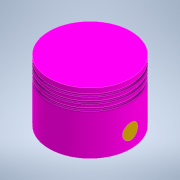
# Autodesk Inventor part: Piston
Saved by Autodesk Inventor 2021 (Build 250183000, 183)
## iProperties
Created: 2021-04-09
Part Number: Piston
Material: Aluminum 6061
Document SubType Name: Modeling
Designer: tommy
Density: 2.7 g/cm^3
Appearance: Magenta
Mass: 463.137 g
Surface Area: 642.196 cm^2
Volume: 171.532 cm^3
bore_dia: 4.000 in
piston_height: 3.000 in
d3: 0.00 deg
wall_thick: 0.250 in
d6: 2.750 in
d7: 0.00 deg
pin_dia: 0.750 in
d11: 1.500 in
d12: 0.750 in
d14: 0.00 deg
ring_depth: 0.100 in
ring_height: 0.150 in
ring_offset: 0.250 in
d19: 3.000 ul
ring_spacing: 0.300 in
Author: tommy
Autodesk Inventor part; units mm, degrees
ref_plane "YZ Plane" through (0, 0, 0) normal (1, 0, 0) x (0, 1, 0)
ref_plane "XZ Plane" through (0, 0, 0) normal (0, 1, 0) x (-1, 0, 0)
ref_plane "XY Plane" through (0, 0, 0) normal (0, 0, 1) x (1, 0, 0)
sketch "Sketch1" plane through (0, 0, 0) normal (0, 1, 0) x (-1, 0, 0)
  circle A0 centre (0, 0) radius 50.8
  dimension "bore_dia" = 101.6
  constraints: 1 centre point, 1 coincident
  measures "bore_dia" diameter of A0
extrude "Extrusion1" add sketch "Sketch1" against normal mid plane 76.2
sketch "Sketch2" plane through (0, -38.1, 0) normal (0, -1, 0) x (1, 0, 0)
  circle A0 centre (0, 0) radius 44.45
  circle A1 centre (0, 0) radius 50.8 projected
  circle A2 centre (0, 0) radius 50.8 projected
  dimension "wall_thick" = 6.35
  constraints: 1 centre point, 1 coincident
  measures "wall_thick" radial gap between concentric circles of A1 A0
extrude "Extrusion2" cut sketch "Sketch2" against normal blind 69.85 contours A0
sketch "Sketch3" plane through (0, 0, 0) normal (1, 0, 0) x (0, 1, 0)
  circle A0 centre (-19.05, 0) radius 9.525
  line L0 (-45.72, 0) -> (7.62, 0) construction
  line L1 (-38.1, -44.45) -> (-38.1, 44.45) construction
  line L2 (0, -115.57) -> (0, 115.57) construction
  point P0 (0, 0)
  dimension "pin_dia" = 19.05
  dimension "d11" = 38.1
  dimension "d12" = 19.05
  constraints: 1 centre point, 1 midpoint
  measures "pin_dia" diameter of A0
  measures "d11" distance between parallel lines of L1 L2
  measures "d12" distance from line of L1 A0.centre
extrude "Extrusion3" cut sketch "Sketch3" along normal through all both and the other way through all
sketch "Sketch4" plane through (0, 0, 0) normal (0, 0, 1) x (1, 0, 0)
  line L0 (50.8, 38.1) -> (-50.8, 38.1) projected
  line L1 (50.8, 38.1) -> (50.8, -38.1) projected
  line L2 (50.8, 31.75) -> (48.26, 31.75)
  line L3 (48.26, 31.75) -> (48.26, 27.94)
  line L4 (48.26, 27.94) -> (50.8, 27.94)
  line L5 (0, -53.34) -> (0, 53.34) projected
  point P0 (0, 0)
  dimension "ring_depth" = 2.54
  dimension "ring_height" = 3.81
  dimension "ring_offset" = 6.35
  constraints: 6 end point, 2 horizontal, 2 point on line, 1 vertical
  measures "ring_depth" distance between parallel lines of L1 L3
  measures "ring_height" distance between parallel lines of L4 L2
  measures "ring_offset" distance between parallel lines of L2 L0
revolve "Revolution1" cut sketch "Sketch4" angle 360 about axis through (0, -10, 0) along (0, 1, 0)
pattern_linear "Rectangular Pattern1" count 3 spacing 7.62 along (0, -1, 0) of "Revolution1"
sketch "Sketch5" plane through (0, 0, 0) normal (1, 0, 0) x (0, 1, 0)
  spline S0 degree 5 poles (-9.525, 0) (-9.525, 0.6718) (-9.5842, 1.3419) (-9.702, 1.9979) (-9.8731, 2.6287) (-10.406, 4.11) (-10.8224, 4.9233) (-11.3102, 5.6469) (-11.8496, 6.2871) (-13.5771, 7.9579) (-14.8799, 8.752) (-16.2472, 9.2671) (-17.648, 9.525) (-20.4517, 9.525) (-21.8536, 9.2669) (-23.2193, 8.7522) (-24.5227, 7.958) (-26.0077, 6.5219) (-26.3305, 6.1698) (-26.6375, 5.7899) (-26.9255, 5.3817) (-27.4836, 4.4629) (-27.7493, 3.9451) (-27.9807, 3.394) (-28.1713, 2.8134) (-28.4169, 1.7825) (-28.4953, 1.3452) (-28.5484, 0.8997) (-28.575, 0.45) (-28.575, -0.45) (-28.5484, -0.8997) (-28.4953, -1.3452) (-28.4169, -1.7825) (-28.1713, -2.8134) (-27.9807, -3.394) (-27.7493, -3.9451) (-27.4836, -4.4629) (-26.9255, -5.3817) (-26.6375, -5.7899) (-26.3305, -6.1698) (-26.0077, -6.5219) (-24.5229, -7.9579) (-23.2201, -8.752) (-21.8528, -9.2671) (-20.452, -9.525) (-17.6483, -9.525) (-16.2464, -9.2669) (-14.8807, -8.7522) (-13.5773, -7.958) (-11.8496, -6.2871) (-11.3102, -5.6469) (-10.8224, -4.9233) (-10.406, -4.11) (-9.8731, -2.6287) (-9.702, -1.9979) (-9.5842, -1.3419) (-9.525, -0.6718) (-9.525, 0) knots 0 0 0 0 0 0 0.045995 0.045995 0.045995 0.045995 0.114362 0.114362 0.114362 0.114362 0.250086 0.250086 0.250086 0.250086 0.38578 0.38578 0.38578 0.38578 0.425457 0.425457 0.425457 0.425457 0.469273 0.469273 0.469273 0.469273 0.500079 0.500079 0.500079 0.500079 0.530886 0.530886 0.530886 0.530886 0.574702 0.574702 0.574702 0.574702 0.614379 0.614379 0.614379 0.614379 0.75006 0.75006 0.75006 0.75006 0.885711 0.885711 0.885711 0.885711 0.954034 0.954034 0.954034 0.954034 1 1 1 1 1 1 projected
  point P0 (0, 0)
  constraints: 1 other
extrude "Extrusion4" add sketch "Sketch5" along normal up to surface separate body round surface about axis through (0, 0, 0) along (0, -1, 0) radius 50.8 far side no
mirror "Mirror1" about plane through (0, 0, 0) normal (1, 0, 0) of "Extrusion4" bodies 2
equation "\"d6\" = piston_height - wall_thick"
equation "\"d12\" = 0.5 * d11"
equation "\"piston_height\" = 76.2"
body "Solid1"
body "Solid2"
